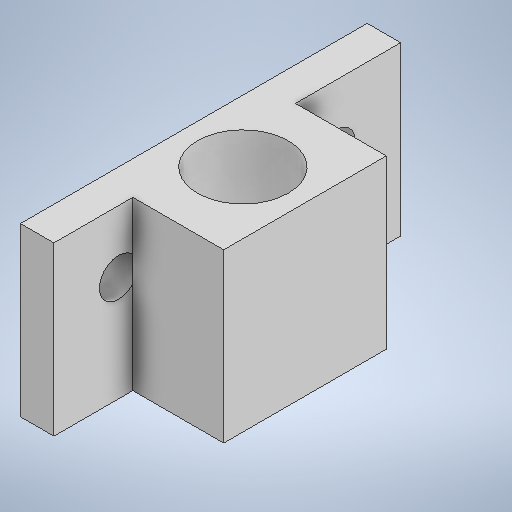
# Autodesk Inventor part: carriage
Saved by Autodesk Inventor 2025.1 (Build 291241000, 241)
## iProperties
Created: 2025-11-11
Part Number: carriage
Material: Generic
Document SubType Name: Modeling
Designer: mukund
Density: 1 g/cm^3
Appearance: Default
Author: mukund
Autodesk Inventor part; units mm, degrees
ref_plane "YZ Plane" through (0, 0, 0) normal (1, 0, 0) x (0, 1, 0)
ref_plane "XZ Plane" through (0, 0, 0) normal (0, 1, 0) x (-1, 0, 0)
ref_plane "XY Plane" through (0, 0, 0) normal (0, 0, 1) x (1, 0, 0)
sketch "Sketch1" plane through (0, 0, 0) normal (0, 1, 0) x (-1, 0, 0)
  line L0 (26, -72.5) -> (-26, -72.5)
  line L1 (-26, -72.5) -> (-26, 72.5)
  line L2 (-26, 72.5) -> (26, 72.5)
  line L3 (26, 72.5) -> (26, -72.5)
  line L4 (26, -72.5) -> (-26, 72.5) construction
  line L5 (-26, -72.5) -> (26, 72.5) construction
  point P0 (0, 0)
  dimension "d0" = 52
  dimension "d1" = 145
  constraints: 12 end point, 2 midpoint, 2 parallel, 1 horizontal, 1 perpendicular
  measures "d0" distance of L1.end L2.end
  measures "d1" distance of L0.end L1.end
extrude "Extrusion1" add sketch "Sketch1" along normal mid plane 70
sketch "Sketch2" plane through (0, 35, 0) normal (0, 1, 0) x (1, 0, 0)
  line L0 (26, -72.5) -> (26, 72.5) projected
  line L1 (26, 72.5) -> (-12, 72.5)
  line L2 (26, 72.5) -> (-26, 72.5) projected
  line L3 (-12, 72.5) -> (-12, 28.5)
  line L4 (-12, 28.5) -> (26, 28.5)
  line L5 (26, 28.5) -> (26, -39.5)
  line L6 (-26, -72.5) -> (26, -72.5) projected
  line L7 (26, -39.5) -> (-12, -39.5)
  line L8 (-12, -39.5) -> (-12, -72.5)
  point P0 (0, 0)
  point P1 (-12, -37.5)
  dimension "d4" = 38
  dimension "d5" = 44
  dimension "d6" = 68
  constraints: 12 end point, 5 point on line, 2 perpendicular, 1 horizontal, 1 vertical
  measures "d4" distance of L0.end L1.end
  measures "d5" distance of L1.end L3.end
  measures "d6" distance of L4.end L5.end
extrude "Extrusion2" cut sketch "Sketch2" against normal blind 70
sketch "Sketch3" plane through (-12, 35, 72.5) normal (1, 0, 0) x (0, 0, -1)
  line L0 (145, 0) -> (0, 0) projected
  line L1 (0, 0) -> (0, -26)
  line L2 (0, 0) -> (0, -70) projected
  line L3 (0, -26) -> (27, -26)
  circle A0 centre (27, -26) radius 8
  line L4 (145, 0) -> (145, -26)
  line L5 (145, 0) -> (145, -70) projected
  line L6 (145, -26) -> (118, -26)
  circle A1 centre (118, -26) radius 8
  point P0 (72.5, -35)
  dimension "d9" = 26
  dimension "d10" = 27
  dimension "d11" = 16
  dimension "d12" = 26
  dimension "d13" = 27
  dimension "d14" = 16
  constraints: 8 end point, 2 centre point, 2 coincident, 2 perpendicular, 2 point on line
  measures "d9" distance of L0.end L1.end
  measures "d10" distance of L1.end L3.end
  measures "d11" diameter of A0
  measures "d12" distance of L0.start L4.end
  measures "d13" distance of L4.end L6.end
  measures "d14" diameter of A1
extrude "Extrusion3" cut sketch "Sketch3" against normal blind 70
sketch "Sketch4" plane through (0, 35, 0) normal (0, 1, 0) x (1, 0, 0)
  line L0 (26, 28.5) -> (26, -39.5) projected
  line L1 (26, -39.5) -> (0, -39.5)
  line L2 (0, -39.5) -> (0, -5.5)
  circle A0 centre (0, -5.5) radius 19
  point P0 (0, 0)
  dimension "d17" = 34
  dimension "d18" = 38
  constraints: 4 end point, 1 centre point, 1 coincident, 1 horizontal, 1 perpendicular
  measures "d17" distance of L1.end L2.end
  measures "d18" diameter of A0
extrude "Extrusion4" cut sketch "Sketch4" against normal blind 70
body "Solid1"
